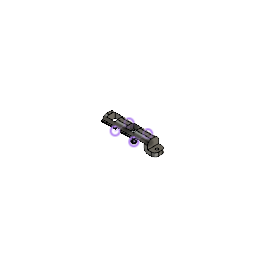
Languette Light FINAL (Autodesk Fusion 360 design; units mm, degrees)
Autodesk Fusion 360 part; units mm, degrees
note: some values were not read from the file. Set by a fixed rule: which face or edge a step refers to.
sketch "Sketch1" plane through (0, 0, 0) normal (0, 0, 1) x (1, 0, 0)
  line L0 (7.5, 7.5) -> (-7.5, 7.5)
  line L1 (-7.5, 7.5) -> (-7.5, -7.5)
  line L2 (-7.5, -7.5) -> (7.5, -7.5)
  line L3 (7.5, -7.5) -> (7.5, 7.5)
  line L4 (7.5, 7.5) -> (-7.5, -7.5) construction
  line L5 (-7.5, 7.5) -> (7.5, -7.5) construction
  dimension "d64_1" = 15
  dimension "d65_1" = 15
  constraint horizontal L0
  constraint perpendicular L0 L1
  constraint parallel L0 L2
  constraint parallel L1 L3
  constraint coincident L4 origin
  constraint coincident L5 origin
  measures "d64_1" distance of L1.end L2.end
  measures "d65_1" distance of L0.end L1.end
sketch "Sketch2" plane through (0, 0, 0) normal (0, 0, 1) x (1, 0, 0)
  line L0 (7.5, -7.5) -> (7.5, 7.5) construction
  line L1 (7.5, 0) -> (12.7, 0) construction
  dimension "d66_1" = 5.2
  constraint midpoint L0 L1.start
  constraint perpendicular L0 L1
  measures "d66_1" distance of L1.start L1.end
sketch "Sketch3" plane through (0, 0, 0) normal (0, 0, 1) x (1, 0, 0)
  line L0 (12.7, 7.5) -> (27.7, 7.5)
  line L1 (27.7, 7.5) -> (27.7, -7.5)
  line L2 (27.7, -7.5) -> (12.7, -7.5)
  line L3 (12.7, -7.5) -> (12.7, 7.5)
  dimension "d67_1" = 15
  dimension "d68_1" = 15
  constraint horizontal L0
  constraint vertical L1
  constraint horizontal L2
  constraint vertical L3
  measures "d67_1" distance of L0.start L0.end
  measures "d68_1" distance of L0.start L2.end
sketch "Sketch4" plane through (0, 0, 0) normal (0, 0, 1) x (1, 0, 0)
  line L0 (27.7, 7.5) -> (27.7, -7.5) construction
  line L1 (27.7, 0) -> (36.7, 0) construction
  dimension "d69_1" = 9
  constraint midpoint L0 L1.start
  constraint perpendicular L0 L1
  measures "d69_1" distance of L1.start L1.end
extrude "Extrude1" add sketch "Sketch1" sketch "Sketch3" along normal blind 2.5 of sketch 2 makes body 1 at (-2.5, 2.5, 0) makes body 2 at (17.7, 2.5, 0)
ref_plane "WorkPlane1" through (0, 0, 2.5) normal (0, 0, 1) x (1, 0, 0)
sketch "Sketch5" plane through (0, 0, 2.5) normal (0, 0, 1) x (1, 0, 0)
  line L0 (0, 0) -> (0, 6) construction
  line L1 (-7.5, 6) -> (37, 6)
  line L2 (37, 6) -> (37, -6)
  line L3 (37, -6) -> (-7.5, -6)
  line L4 (-7.5, -6) -> (-7.5, 6)
  dimension "d73_1" = 6
  constraint coincident L0.start origin
  constraint vertical L0
  constraint horizontal L1
  constraint vertical L2
  constraint horizontal L3
  constraint vertical L4
  measures "d73_1" distance of L0.start L0.end
extrude "Extrude2" add sketch "Sketch5" along normal blind 4 bodies 1 2
ref_plane "WorkPlane2" through (37, 0, 0) normal (1, 0, 0) x (0, 1, 0)
ref_plane "WorkPlane3" through (14.75, 0, -1.7) normal (0, 0, 1) x (1, 0, 0)
sketch "Sketch6" plane through (37, 0, 0) normal (1, 0, 0) x (0, 1, 0)
  line L0 (-6, 2.5) -> (6, 2.5)
  line L1 (6, 2.5) -> (6, 6.5)
  line L2 (6, 6.5) -> (-6, 6.5)
  line L3 (-6, 6.5) -> (-6, 2.5)
  line L4 (-6, 6.5) -> (6, 6.5)
  line L5 (6, 6.5) -> (6, -1.7)
  line L6 (6, -1.7) -> (-6, -1.7)
  line L7 (-6, -1.7) -> (-6, 6.5)
  dimension "d78_1" = 12
  dimension "d79_1" = 8.2
  constraint horizontal L4
  constraint vertical L5
  constraint horizontal L6
  constraint vertical L7
  constraint coincident L2.end L3.start
  measures "d78_1" distance of L2.end L1.end
  measures "d79_1" distance of L2.end L6.end
extrude "Extrude3" add sketch "Sketch6" along normal blind 4 bodies 1
sketch "Sketch7" plane through (0, 0, -1.7) normal (0, 0, 1) x (1, 0, 0)
  line L0 (37, -6) -> (49, -6)
  line L1 (49, -6) -> (49, 6)
  line L2 (49, 6) -> (37, 6)
  line L3 (37, 6) -> (37, -6)
  dimension "d82_1" = 12
  constraint horizontal L0
  constraint vertical L1
  constraint horizontal L2
  constraint vertical L3
  measures "d82_1" distance of L0.start L0.end
extrude "Extrude4" add sketch "Sketch7" against normal blind 4 bodies 1
sketch "Sketch8" plane through (0, 0, -1.7) normal (0, 0, 1) x (-1, 0, 0)
  line L0 (-41, -6) -> (-41, 6)
  line L1 (-41, 6) -> (-49, 6)
  line L2 (-49, 6) -> (-49, -6)
  line L3 (-49, -6) -> (-41, -6)
  circle A0 centre (-45.3458, 0.0801) radius 1.35
  dimension "d85_1" = 2.7
  measures "d85_1" diameter of A0
extrude "Extrude5" cut sketch "Sketch8" against normal blind 8 contours A0 bodies 1
fillet "Fillet1" radius 4 1 edges at (16.75, -6, 6.5) on bodies 1
fillet "Fillet2" radius 4 1 edges at (16.75, 6, 6.5) on bodies 1
fillet "Fillet3" radius 4 1 edges at (49, 6, -3.7) on bodies 1
fillet "Fillet4" radius 4 1 edges at (49, -6, -3.7) on bodies 1
fillet "Fillet5" radius 4 1 edges at (37, 0, -5.7) on bodies 1
fillet "Fillet6" radius 1.5 6 edges at (20.2, 7.5, 0) (12.7, 0, 0) (20.2, -7.5, 0) (0, 7.5, 0) (-7.5, 0, 0) (0, -7.5, 0) 2 faces at (-2.5, 2.5, 0) (17.7, 2.5, 0) on bodies 1 2
sketch "Sketch9" plane through (0, 0, -1.7) normal (0, 0, 1) x (1, 0, 0)
  line L0 (-6, 6) -> (6, -6) construction
sketch "Sketch10" plane through (0, 0, 0) normal (0, 0, -1) x (1, 0, 0)
  line L0 (26.2, 6) -> (14.2, 6)
  line L1 (14.2, 6) -> (14.2, -6)
  line L2 (14.2, -6) -> (26.2, -6)
  line L3 (26.2, -6) -> (26.2, 6)
  line L4 (14.2, -6) -> (26.2, 6) construction
  constraint coincident L1.end L2.start
  constraint coincident L0.start L3.end
sketch "Sketch11" plane through (0, 0, 0) normal (0, 0, -1) x (1, 0, 0)
  line L0 (26.2, 6) -> (14.2, 6)
  line L1 (14.2, 6) -> (14.2, -6)
  line L2 (14.2, -6) -> (26.2, -6)
  line L3 (26.2, -6) -> (26.2, 6)
  line L4 (24.7, -4.5) -> (15.7, -4.5)
  line L5 (15.7, -4.5) -> (15.7, 4.5)
  line L6 (15.7, 4.5) -> (24.7, 4.5)
  line L7 (24.7, 4.5) -> (24.7, -4.5)
  line L8 (24.7, -4.5) -> (15.7, 4.5) construction
  line L9 (15.7, -4.5) -> (24.7, 4.5) construction
  line L10 (14.2, -6) -> (26.2, 6)
  point P0 (20.2, 0)
  dimension "d119" = 9
  dimension "d120" = 9
  constraint horizontal L4
  constraint perpendicular L4 L5
  constraint parallel L4 L6
  constraint parallel L5 L7
  constraint coincident L8 P0
  constraint coincident L9 P0
  constraint midpoint P0 L10
  measures "d119" distance of L5.end L6.end
  measures "d120" distance of L4.end L5.end
sketch "Sketch12" plane through (0, 0, 0) normal (0, 0, -1) x (1, 0, 0)
  line L0 (6, -6) -> (6, 6)
  line L1 (6, 6) -> (-6, 6)
  line L2 (-6, 6) -> (-6, -6)
  line L3 (-6, -6) -> (6, -6)
  line L4 (4.5, -4.5) -> (-4.5, -4.5)
  line L5 (-4.5, -4.5) -> (-4.5, 4.5)
  line L6 (-4.5, 4.5) -> (4.5, 4.5)
  line L7 (4.5, 4.5) -> (4.5, -4.5)
  line L8 (4.5, -4.5) -> (-4.5, 4.5) construction
  line L9 (-4.5, -4.5) -> (4.5, 4.5) construction
  dimension "d121" = 9
  dimension "d122" = 9
  constraint horizontal L4
  constraint perpendicular L4 L5
  constraint parallel L4 L6
  constraint parallel L5 L7
  constraint coincident L8 origin
  constraint coincident L9 origin
  measures "d121" distance of L5.end L6.end
  measures "d122" distance of L4.end L5.end
ref_plane "WorkPlane4" through (-7.5, 7.5, 1.5) normal (-1, 0, 0) x (0, -1, 0)
extrude "Extrude6" cut sketch "Sketch12" against normal blind 10 contours L4 L5 L6 L7 bodies 1
extrude "Extrude7" cut sketch "Sketch11" against normal blind 10 contours L5 L6 L10 | L4 L7 L10 bodies 1
